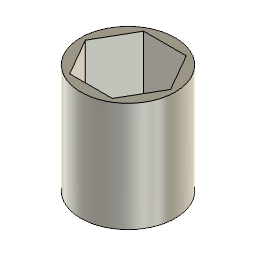
penplotter_attachment_hole v1 (Autodesk Fusion 360 design; units mm, degrees)
Autodesk Fusion 360 part; units mm, degrees
sketch "スケッチ1" plane through (0, 0, 0) normal (0, 0, 1) x (1, 0, 0)
  circle A0 centre (0, 0) radius 3.45
  line L0 (3.1177, 0) -> (1.5588, 2.7)
  line L1 (1.5588, 2.7) -> (-1.5588, 2.7)
  line L2 (-1.5588, 2.7) -> (-3.1177, 0)
  line L3 (-3.1177, 0) -> (-1.5588, -2.7)
  line L4 (-1.5588, -2.7) -> (1.5588, -2.7)
  line L5 (1.5588, -2.7) -> (3.1177, 0)
  dimension "d1" = 6.9
  dimension "d2" = 5.4
  constraint coincident A0.centre origin
  measures "d1" diameter of A0
  measures "d2" distance of L1 L4
extrude "押し出し1" add sketch "スケッチ1" along normal blind 8
